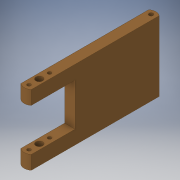
# Autodesk Inventor part: GripperArm
Saved by Autodesk Inventor 2019 (Build 230136000, 136)
## iProperties
Created: 2019-10-02
Part Number: GripperArm
Material: Generic
Document SubType Name: Modeling
Designer: james
Density: 1 g/cm^3
Appearance: Default(1)
Author: james
Autodesk Inventor part; units mm, degrees
ref_plane "YZ Plane" through (0, 0, 0) normal (1, 0, 0) x (0, 1, 0)
ref_plane "XZ Plane" through (0, 0, 0) normal (0, 1, 0) x (-1, 0, 0)
ref_plane "XY Plane" through (0, 0, 0) normal (0, 0, 1) x (1, 0, 0)
sketch "Sketch1" plane through (0, 0, 0) normal (0, 1, 0) x (-1, 0, 0)
  line L0 (-6.8943, 36.0441) -> (-6.8943, -70.6359)
  line L1 (8.3457, -70.6359) -> (8.3457, 36.0441)
  arc A0 (8.3457, 36.0441) -> (-6.8943, 36.0441) centre (0.7257, 36.0441) ccw
  arc A1 (-6.8943, -70.6359) -> (8.3457, -70.6359) centre (0.7257, -70.6359) ccw
  point P0 (0, 0)
  dimension "d2" = 15.24
  dimension "d4" = 7.62
  dimension "d5" = 15.24
  dimension "d6" = 7.62
  dimension "d8" = 106.68
  dimension "d9" = 15.24
  constraints: 4 end point, 4 point on circle, 2 centre point, 1 parallel
  measures "d2" diameter of A1
  measures "d4" distance from line of L0 A1.centre
  measures "d5" diameter of A0
  measures "d6" distance from line of L0 A0.centre
  measures "d8" distance of A1.centre A0.centre
  measures "d9" distance between parallel lines of L0 L1
extrude "Extrusion1" add sketch "Sketch1" along normal blind 64.77
sketch "Sketch2" plane through (0, 64.77, 0) normal (0, 1, 0) x (1, 0, 0)
  line L0 (6.8943, -36.0441) -> (6.8943, 70.6359) projected
  arc A0 (-8.3457, -36.0441) -> (6.8943, -36.0441) centre (-0.7257, -36.0441) ccw projected
  point P0 (0, 0)
  point P1 (-0.7257, -39.2191)
  point P2 (-0.7257, -29.6941)
  point P3 (-0.7257, -20.1691)
  dimension "d16" = 7.62
  dimension "d47" = 0
  dimension "d48" = 0
  dimension "d49" = 6.35
  dimension "d50" = 9.525
  dimension "d51" = 9.525
  measures "d16" distance from line of L0 point (-0.726, -39.219)
  measures "d47" horizontal distance of point (-0.726, -29.694) point (-0.726, -39.219)
  measures "d48" horizontal distance of point (-0.726, -20.169) point (-0.726, -29.694)
  measures "d49" distance of point (-0.726, -29.694) A0.centre
  measures "d50" distance of point (-0.726, -20.169) point (-0.726, -29.694)
  measures "d51" distance of point (-0.726, -29.694) point (-0.726, -39.219)
hole "Hole1" at (-0.7257, 64.77, 39.2191) at (-0.7257, 64.77, 29.6941) at (-0.7257, 64.77, 20.1691) direction (0, -1, 0) diameter 3.2766 end through all clearance for "Flat Head Machine Screw (82)" size "#4" standard "Ansi Unified Screw Threads"
sketch "Sketch3" plane through (0, 64.77, 0) normal (0, 1, 0) x (1, 0, 0)
  line L0 (-8.3457, 70.6359) -> (-8.3457, -36.0441) projected
  arc A0 (6.8943, 70.6359) -> (-8.3457, 70.6359) centre (-0.7257, 70.6359) ccw projected
  point P0 (0, 0)
  point P1 (-0.7257, 73.8109)
  dimension "d25" = 7.62
  dimension "d43" = 3.175
  measures "d25" distance from line of point (-0.726, 73.811) L0
  measures "d43" distance of A0.centre point (-0.726, 73.811)
hole "Hole2" at (-0.7257, 64.77, -73.8109) direction (0, -1, 0) diameter 3.81 end through all clearance for "Flat Head Machine Screw (82)" size "#6" standard "Ansi Unified Screw Threads"
sketch "Sketch4" plane through (0, 64.77, 0) normal (0, 1, 0) x (1, 0, 0)
  line L0 (39.3169, 103.6547) -> (4.1003, 103.6547)
  line L1 (4.1003, 103.6547) -> (4.1003, -56.0742)
  line L2 (4.1003, -56.0742) -> (39.3169, -56.0742)
  line L3 (39.3169, -56.0742) -> (39.3169, 103.6547)
  line L4 (-5.5517, 100.2529) -> (-25.9242, 100.2529)
  line L5 (-25.9242, 100.2529) -> (-25.9242, -57.002)
  line L6 (-25.9242, -57.002) -> (-5.5517, -57.002)
  line L7 (-5.5517, -57.002) -> (-5.5517, 100.2529)
  line L8 (-8.3457, 70.6359) -> (-8.3457, -36.0441) projected
  line L9 (6.8943, -36.0441) -> (6.8943, 70.6359) projected
  point P0 (0, 0)
  dimension "d34" = 2.794
  dimension "d35" = 2.794
  constraints: 16 end point, 4 parallel, 2 horizontal, 2 perpendicular
  measures "d34" distance between parallel lines of L8 L7
  measures "d35" distance between parallel lines of L9 L1
extrude "Extrusion2" cut sketch "Sketch4" against normal blind 101.6
sketch "Sketch5" plane through (4.1003, 64.77, 41.941) normal (1, 0, 0) x (0, 0, -1)
  line L0 (-34.9815, -12.7) -> (40.64, -12.7)
  line L1 (40.64, -12.7) -> (40.64, -52.07)
  line L2 (40.64, -52.07) -> (-34.9815, -52.07)
  line L3 (-34.9815, -52.07) -> (-34.9815, -12.7)
  line L4 (0, -64.77) -> (0, 0) projected
  line L5 (0, 0) -> (118.4739, 0) projected
  line L6 (118.4739, -64.77) -> (0, -64.77) projected
  point P0 (41.941, -64.77)
  dimension "d38" = 40.64
  dimension "d39" = 12.7
  dimension "d40" = 12.7
  constraints: 8 end point, 2 parallel, 1 horizontal, 1 perpendicular
  measures "d38" distance between parallel lines of L1 L4
  measures "d39" distance between parallel lines of L5 L0
  measures "d40" distance between parallel lines of L6 L2
extrude "Extrusion3" cut sketch "Sketch5" against normal blind 25.4
sketch "Sketch6" plane through (0, 64.77, 0) normal (0, 1, 0) x (1, 0, 0)
  circle A0 centre (-0.7257, -29.6941) radius 1.6383 projected
  circle A1 centre (-0.7257, -29.6941) radius 3.175
  point P0 (0, 0)
  dimension "d44" = 6.35
  constraints: 1 centre point, 1 coincident
  measures "d44" diameter of A1
extrude "Extrusion4" cut sketch "Sketch6" against normal blind 101.6
body "Solid1"
